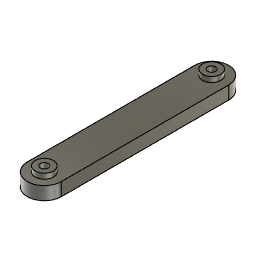
BarreAutre v2 (Autodesk Fusion 360 design; units mm, degrees)
Autodesk Fusion 360 part; units mm, degrees
sketch "Esquisse1" plane through (0, 0, 0) normal (0, 0, 1) x (1, 0, 0)
  circle A0 centre (0, 0) radius 6.5
  circle A1 centre (0, 64) radius 6.5
  line L0 (0, 64) -> (0, 0)
  line L1 (0, 64) -> (6.5, 64)
  line L2 (0, 64) -> (-6.5, 64)
  line L3 (0, 0) -> (6.5, 0)
  line L4 (0, 0) -> (-6.5, 0)
  line L5 (6.5, 64) -> (6.5, 0)
  line L6 (-6.5, 64) -> (-6.5, 0)
  circle A2 centre (0, 64) radius 1.5
  circle A3 centre (0, 0) radius 1.5
  dimension "d1" = 13
  dimension "d2" = 13
  dimension "d3" = 64
  dimension "d4" = 3
  dimension "d5" = 3
  constraint coincident A0.centre L0.end
  constraint coincident A1.centre L0.start
  constraint vertical L0
  constraint coincident A1 L1.end
  constraint perpendicular L0 L1
  constraint coincident A1 L2.end
  constraint perpendicular L0 L2
  constraint coincident A0 L3.end
  constraint perpendicular L0 L3
  constraint coincident A0 L4.end
  constraint perpendicular L0 L4
  measures "d1" diameter of A0
  measures "d2" diameter of A1
  measures "d3" distance of A1.centre A0.centre
  measures "d4" diameter of A2
  measures "d5" diameter of A3
extrude "Extrusion1" add sketch "Esquisse1" along normal blind 5 contours A0 L3 L4 A3 | A0 A1 L0 L6 | A0 L0 L4 A3 | A0 L0 L3 A3 | A0 A1 L0 L5 | A1 L0 L2 A2 | A1 L1 L2 A2 | A1 L0 L1 A2
sketch "Esquisse2" plane through (0, 0, 5) normal (0, 0, 1) x (-1, 0, 0)
  circle A0 centre (0, 0) radius 1.5
  circle A1 centre (0, -64) radius 1.5
  arc A2 (-6.5, -64) -> (6.5, -64) centre (0, -64) ccw
  line L0 (6.5, -64) -> (6.5, 0)
  arc A3 (6.5, 0) -> (-6.5, 0) centre (0, 0) ccw
  line L1 (-6.5, 0) -> (-6.5, -64)
  circle A4 centre (0, -64) radius 3.5
  circle A5 centre (0, -64) radius 1.5
  circle A6 centre (0, 0) radius 1.5
  circle A7 centre (0, 0) radius 3.5
  dimension "d8" = 3
  dimension "d9" = 7
  dimension "d10" = 3
  dimension "d11" = 7
  constraint concentric A1 A4
  constraint concentric A4 A5
  constraint concentric A0 A6
  constraint coincident A0.centre A3.centre
  measures "d8" diameter of A6
  measures "d9" diameter of A7
  measures "d10" diameter of A5
  measures "d11" diameter of A4
extrude "Extrusion2" add sketch "Esquisse2" along normal blind 2 contours A4 | A7
